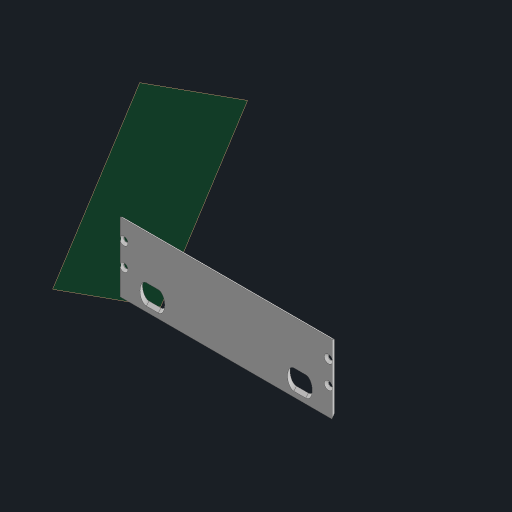
# Autodesk Inventor part: front
Saved by Autodesk Inventor 2023 (Build 270158000, 158)
## iProperties
Created: 2024-04-25
Part Number: front
Material: Generic
Document SubType Name: Modeling
Designer: szymo
Density: 1 g/cm^3
Appearance: Default
Author: szymo
Autodesk Inventor part; units mm, degrees
ref_plane "YZ Plane" through (0, 0, 0) normal (1, 0, 0) x (0, 1, 0)
ref_plane "XZ Plane" through (0, 0, 0) normal (0, 1, 0) x (-1, 0, 0)
ref_plane "XY Plane" through (0, 0, 0) normal (0, 0, 1) x (1, 0, 0)
ref_plane "Work Plane1" through (0, 4.7283, -22.9522) normal (-1, 0, 0) x (0, -0.8411785, 0.5407576)
sketch "Sketch1" plane through (0, 4.7283, -22.9522) normal (-1, 0, 0) x (0, -0.8411785, 0.5407576)
  arc A0 (-58.25, -16.75) -> (-61.5, -13.5) centre (-58.25, -13.5) ccw projected
  line L0 (-58.25, -16.75) -> (-33, -16.75) projected
  circle A1 centre (-33, -13.5) radius 3.25 projected
  line L1 (-33, -16.75) -> (61.5, -16.75) projected
  line L2 (61.5, -16.75) -> (61.5, -12.25) projected
  line L3 (61.5, -12.25) -> (16.3889, 16.75) projected
  line L4 (16.3889, 16.75) -> (-61.5, 16.75) projected
  line L5 (-61.5, 16.75) -> (-61.5, -13.5) projected
  line L6 (61.5, -12.25) -> (61.5, -16.75) projected
  line L7 (61.5, -16.75) -> (65.5, -16.75) projected
  line L8 (65.5, -16.75) -> (65.5, -20.25) projected
  line L9 (65.5, -20.25) -> (79.5, -20.25) projected
  line L10 (79.5, -20.25) -> (65.5, -11.25) projected
  line L11 (65.5, -11.25) -> (65.5, -12.25) projected
  line L12 (65.5, -12.25) -> (61.5, -12.25) projected
  line L13 (16.3889, 16.75) -> (16.3889, 18.75) projected
  line L14 (14.3494, 18.75) -> (16.3889, 18.75) projected
  line L15 (65.5, -12.25) -> (13.8896, 20.9281)
  line L16 (16.3889, 16.75) -> (16.3889, 19.3214)
  constraints: 4 end point, 1 parallel, 1 point on line, 1 vertical, 1 vertical alignment
ref_plane "Work Plane2" through (178, -56.0619, -70.2985) normal (1, 0, 0) x (0, 0.8411785, -0.5407576)
extrude "Extrusion1" add sketch "Sketch1" against normal up to surface (178 mm away) contours L13 L16 L15 L12 L3
sketch "Sketch2" plane through (0, -56.9932, 2.163) normal (0, 0, 1) x (1, 0, 0)
  circle A0 centre (3, 23.0218) radius 2.5 projected
  circle A1 centre (3, 42.3361) radius 2.5 projected
  line L0 (0, 3.3647) -> (0, 56.9932) projected
  line L1 (0, 3.3647) -> (6, 3.3647) projected
  line L2 (6, 56.9932) -> (6, 3.3647) projected
  line L3 (0, 56.9932) -> (6, 56.9932) projected
  circle A2 centre (175, 23.0218) radius 2.5 projected
  circle A3 centre (175, 42.3361) radius 2.5 projected
  line L4 (178, 3.3647) -> (178, 56.9932) projected
  line L5 (178, 56.9932) -> (172, 56.9932) projected
  line L6 (172, 56.9932) -> (172, 3.3647) projected
  line L7 (178, 3.3647) -> (172, 3.3647) projected
  constraints: 4 coincident
hole "Hole1" at (3, -14.6571, 2.163) at (3, -33.9713, 2.163) at (175, -33.9713, 2.163) at (175, -14.6571, 2.163) direction (0, 0, -1) diameter 3.6 end through all countersink diameter 7 countersink angle 90 clearance for "Countersunk Flat Head Screw ISO 2009/7046" size "M3" standard "ISO"
ref_plane "Work Plane3" through (22, -30.5397, -9.0869) normal (0, -0.7712334, 0.6365525) x (1, 0, 0)
sketch "Sketch3" plane through (22, -30.5397, -9.0869) normal (0, -0.7712334, 0.6365525) x (1, 0, 0)
  line L0 (-9.9215, 5.4518) -> (-9.9215, -5.4534)
  spline S0 degree 3 poles (-9.9215, -5.4534) (-9.9222, -5.5772) (-9.8204, -5.8209) (-9.5772, -5.9222) (-9.4534, -5.9215) knots 0 0 0 0 0.5 1 1 1 1
  line L1 (-9.4534, -5.9215) -> (19.4534, -5.9215)
  spline S1 degree 3 poles (19.4534, -5.9215) (19.5775, -5.9222) (19.8219, -5.82) (19.9222, -5.5758) (19.9215, -5.4518) knots 0 0 0 0 0.5 1 1 1 1
  line L2 (19.9215, -5.4518) -> (19.9215, 5.4534)
  spline S2 degree 3 poles (19.9215, 5.4534) (19.9222, 5.5775) (19.82, 5.8219) (19.5758, 5.9222) (19.4518, 5.9215) knots 0 0 0 0 0.5 1 1 1 1
  line L3 (19.4518, 5.9215) -> (-9.4534, 5.9215)
  spline S3 degree 3 poles (-9.4534, 5.9215) (-9.5775, 5.9222) (-9.8219, 5.82) (-9.9222, 5.5758) (-9.9215, 5.4518) knots 0 0 0 0 0.5 1 1 1 1
  circle A0 centre (-8.3791, -4.3791) radius 0.5
  circle A1 centre (-8.3791, 4.3791) radius 0.5
  circle A2 centre (18.3791, 4.3791) radius 0.5
  circle A3 centre (18.3791, -4.3791) radius 0.5
  arc A4 (5.2617, -1.4512) -> (5.1811, -1.5218) centre (5.2771, -1.55) ccw
  arc A5 (5.1811, 1.5218) -> (5.1811, -1.5218) centre (0, 0) ccw
  arc A6 (5.1811, 1.5218) -> (5.2617, 1.4512) centre (5.2771, 1.55) ccw
  arc A7 (5.2617, 1.4512) -> (5.3414, 1.519) centre (5.2463, 1.55) ccw
  arc A8 (5.3414, -1.519) -> (5.3414, 1.519) centre (10, 0) ccw
  arc A9 (5.3414, -1.519) -> (5.2617, -1.4512) centre (5.2463, -1.55) ccw
  line L4 (143.9215, 5.4518) -> (143.9215, -5.4534)
  spline S4 degree 3 poles (143.4534, 5.9215) (143.5775, 5.9222) (143.8219, 5.82) (143.9222, 5.5758) (143.9215, 5.4518) knots 0 0 0 0 0.5 1 1 1 1
  line L5 (114.5482, 5.9215) -> (143.4534, 5.9215)
  spline S5 degree 3 poles (114.0785, 5.4534) (114.0778, 5.5775) (114.18, 5.8219) (114.4242, 5.9222) (114.5482, 5.9215) knots 0 0 0 0 0.5 1 1 1 1
  line L6 (114.0785, -5.4518) -> (114.0785, 5.4534)
  spline S6 degree 3 poles (114.5466, -5.9215) (114.4225, -5.9222) (114.1781, -5.82) (114.0778, -5.5758) (114.0785, -5.4518) knots 0 0 0 0 0.5 1 1 1 1
  line L7 (143.4534, -5.9215) -> (114.5466, -5.9215)
  spline S7 degree 3 poles (143.9215, -5.4534) (143.9222, -5.5772) (143.8204, -5.8209) (143.5772, -5.9222) (143.4534, -5.9215) knots 0 0 0 0 0.5 1 1 1 1
  circle A10 centre (142.3791, -4.3791) radius 0.5
  circle A11 centre (142.3791, 4.3791) radius 0.5
  circle A12 centre (115.6209, 4.3791) radius 0.5
  circle A13 centre (115.6209, -4.3791) radius 0.5
  arc A14 (128.8189, -1.5218) -> (128.7383, -1.4512) centre (128.7229, -1.55) ccw
  arc A15 (128.7383, -1.4512) -> (128.6586, -1.519) centre (128.7537, -1.55) ccw
  arc A16 (128.6586, 1.519) -> (128.6586, -1.519) centre (124, 0) ccw
  arc A17 (128.6586, 1.519) -> (128.7383, 1.4512) centre (128.7537, 1.55) ccw
  arc A18 (128.7383, 1.4512) -> (128.8189, 1.5218) centre (128.7229, 1.55) ccw
  arc A19 (128.8189, -1.5218) -> (128.8189, 1.5218) centre (134, 0) ccw
  circle A20 centre (10, 0) radius 5.4
  circle A21 centre (124, 0) radius 5.4
  line L8 (0, 5.4) -> (10, 5.4)
  line L9 (10, -5.4) -> (0, -5.4)
  line L10 (124, 5.4) -> (134, 5.4)
  line L11 (134, -5.4) -> (124, -5.4)
  point P0 (-22, 26.4483)
  dimension "d9" = 10.8
  dimension "d10" = 10.8
  constraints: 8 end point, 8 point on circle, 4 point on line, 3 tangent, 2 centre point, 2 coincident
  measures "d9" diameter of A20
  measures "d10" diameter of A21
extrude "Extrusion2" cut sketch "Sketch3" along normal blind 78.25 contours A9 A8 A7 A6 A5 A20 A4 | A4 A5 A20 A6 A7 A8 A9 | A20 L9 A5 | A5 A20 | A5 L8 A20 | A19 A21 A18 A17 A16 A15 A14 | A14 A15 A16 A17 A18 A19 A21 | A21 A19 | A19 L11 A21 | A19 A21 L10
body "Solid1"
